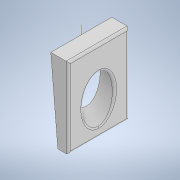
# Autodesk Inventor part: waterHeaterVent-V02
Saved by Autodesk Inventor 2021.1 (Build 251245010, 245A)
## iProperties
Created: 2020-10-25
Part Number: waterHeaterVent-V02
Material: Generic
Document SubType Name: Modeling
Designer: robst
Density: 1 g/cm^3
Appearance: Default
Author: robst
Autodesk Inventor part; units mm, degrees
ref_plane "YZ Plane" through (0, 0, 0) normal (1, 0, 0) x (0, 1, 0)
ref_plane "XZ Plane" through (0, 0, 0) normal (0, 1, 0) x (-1, 0, 0)
sketch "Sketch1" plane through (0, 0, 0) normal (0, 0, 1) x (1, 0, 0)
  line L0 (0, 0) -> (5.1111, -58.42)
  line L1 (0, -70.104) -> (0, 11.684) projected
  line L2 (0, 0) -> (12.7, 0)
  line L3 (12.7, 0) -> (12.7, -58.42)
  line L4 (5.1111, -58.42) -> (12.7, -58.42)
  dimension "d0" = 5
  dimension "d1" = 12.7
  dimension "d3" = 58.42
  constraints: 8 end point, 2 horizontal, 1 vertical
  measures "d0" angle of L0 L1
  measures "d1" distance of L0.start L2.end
  measures "d3" distance of L2.end L3.end
extrude "Extrusion1" add sketch "Sketch1" along normal mid plane 44.45
ref_plane "Work Plane1" through (12.7, -58.42, 0) normal (0.7071, -0.7071, 0) x (0, 0, 1)
sketch "Sketch2" plane through (12.7, -58.42, 0) normal (0.7071, -0.7071, 0) x (0, 0, 1)
  line L0 (22.225, 0) -> (22.225, -41.3092) projected
  line L1 (22.225, -41.3092) -> (-22.225, -41.3092) projected
  line L2 (-22.225, -41.3092) -> (-22.225, 0) projected
  line L3 (-22.225, 0) -> (22.225, 0) projected
  circle A0 centre (0, -15.9092) radius 11.43
  point P0 (0, -32.3289)
  dimension "d7" = 22.86
  dimension "d10" = 25.4
  constraints: 1 centre point
  measures "d7" diameter of A0
  measures "d10" distance from line of A0.centre L1
extrude "Extrusion2" cut sketch "Sketch2" against normal through all contours A0
sketch "Sketch3" plane through (5.1111, -58.42, -22.225) normal (-0.9962, -0.0872, 0) x (0, 0, 1)
  line L0 (0, 0) -> (0, 58.6432) construction
  line L1 (0, 7.62) -> (44.45, 7.62) construction
  line L2 (44.45, 58.6432) -> (44.45, 0) construction
  line L3 (0, 0) -> (44.45, 0) construction
  line L4 (17.7759, 11.43) -> (15.1515, 3.81)
  line L5 (15.1515, 3.81) -> (14.0585, 3.81)
  line L6 (14.0585, 3.81) -> (11.4341, 11.43)
  line L7 (11.4341, 11.43) -> (12.5209, 11.43)
  line L8 (12.5209, 11.43) -> (14.6328, 5.1006)
  line L9 (14.6328, 5.1006) -> (16.7447, 11.43)
  line L10 (16.7447, 11.43) -> (17.7759, 11.43)
  line L11 (21.166, 6.6814) -> (18.2822, 6.6814)
  line L12 (18.2822, 6.6814) -> (18.2822, 7.6077)
  line L13 (18.2822, 7.6077) -> (21.166, 7.6077)
  line L14 (21.166, 7.6077) -> (21.166, 6.6814)
  spline S0 degree 2 poles (26.9211, 7.62) (26.9211, 5.5699) (25.7293, 3.6494) (24.4882, 3.6494) knots 0 0 0 1 2 2 2
  spline S1 degree 2 poles (24.4882, 3.6494) (23.2284, 3.6494) (22.049, 5.6069) (22.049, 7.6138) knots 0 0 0 1 2 2 2
  spline S2 degree 2 poles (22.049, 7.6138) (22.049, 9.6763) (23.2408, 11.5844) (24.4882, 11.5844) knots 0 0 0 1 2 2 2
  spline S3 degree 2 poles (24.4882, 11.5844) (25.7417, 11.5844) (26.9211, 9.6084) (26.9211, 7.62) knots 0 0 0 1 2 2 2
  spline S4 degree 2 poles (25.612, 5.2982) (25.7602, 5.6749) (25.8837, 6.8358) (25.8837, 7.62) knots 0 0 0 1 2 2 2
  spline S5 degree 2 poles (25.8837, 7.62) (25.8837, 8.4042) (25.7602, 9.559) (25.6058, 9.948) knots 0 0 0 1 2 2 2
  spline S6 degree 2 poles (25.6058, 9.948) (25.4515, 10.337) (24.9142, 10.7384) (24.4882, 10.7384) knots 0 0 0 1 2 2 2
  spline S7 degree 2 poles (24.4882, 10.7384) (24.0621, 10.7384) (23.5125, 10.337) (23.3519, 9.9356) knots 0 0 0 1 2 2 2
  spline S8 degree 2 poles (23.3519, 9.9356) (23.1976, 9.5466) (23.0864, 8.361) (23.0864, 7.6138) knots 0 0 0 1 2 2 2
  spline S9 degree 2 poles (23.0864, 7.6138) (23.0864, 6.8111) (23.1852, 5.7366) (23.3458, 5.3167) knots 0 0 0 1 2 2 2
  spline S10 degree 2 poles (23.3458, 5.3167) (23.494, 4.9215) (24.0435, 4.4954) (24.4882, 4.4954) knots 0 0 0 1 2 2 2
  spline S11 degree 2 poles (24.4882, 4.4954) (24.9081, 4.4954) (25.4576, 4.8968) (25.612, 5.2982) knots 0 0 0 1 2 2 2
  line L15 (32.596, 3.81) -> (27.8968, 3.81)
  line L16 (27.8968, 3.81) -> (27.8968, 4.8906)
  spline S12 degree 2 poles (27.8968, 4.8906) (28.4031, 5.3661) (29.3047, 6.2491) (29.7369, 6.7246) knots 0 0 0 1 2 2 2
  spline S13 degree 2 poles (29.7369, 6.7246) (30.6076, 7.6818) (31.2436, 8.8303) (31.2436, 9.4416) knots 0 0 0 1 2 2 2
  spline S14 degree 2 poles (31.2436, 9.4416) (31.2436, 9.7627) (31.046, 10.2444) (30.867, 10.3988) knots 0 0 0 1 2 2 2
  spline S15 degree 2 poles (30.867, 10.3988) (30.6879, 10.5531) (30.2186, 10.7075) (29.9345, 10.7075) knots 0 0 0 1 2 2 2
  spline S16 degree 2 poles (29.9345, 10.7075) (29.6628, 10.7075) (29.1071, 10.5717) (28.8539, 10.4667) knots 0 0 0 1 2 2 2
  spline S17 degree 2 poles (28.8539, 10.4667) (28.6378, 10.3802) (28.2364, 10.1332) (28.1129, 10.0468) knots 0 0 0 1 2 2 2
  line L17 (28.1129, 10.0468) -> (28.0573, 10.0468)
  line L18 (28.0573, 10.0468) -> (28.0573, 11.1336)
  spline S18 degree 2 poles (28.0573, 11.1336) (28.3723, 11.288) (29.5023, 11.5906) (30.0086, 11.5906) knots 0 0 0 1 2 2 2
  spline S19 degree 2 poles (30.0086, 11.5906) (31.0769, 11.5906) (32.2811, 10.4605) (32.2811, 9.4972) knots 0 0 0 1 2 2 2
  spline S20 degree 2 poles (32.2811, 9.4972) (32.2811, 9.0464) (32.0711, 8.2931) (31.8859, 7.972) knots 0 0 0 1 2 2 2
  spline S21 degree 2 poles (31.8859, 7.972) (31.7006, 7.6385) (31.1634, 6.984) (30.867, 6.669) knots 0 0 0 1 2 2 2
  spline S22 degree 2 poles (30.867, 6.669) (30.3853, 6.1442) (29.2059, 5.0203) (28.8539, 4.693) knots 0 0 0 1 2 2 2
  line L19 (28.8539, 4.693) -> (32.596, 4.693)
  line L20 (32.596, 4.693) -> (32.596, 3.81)
  point P0 (22.225, 58.6432)
  dimension "d12" = 7.62
  constraints: 2 end point, 2 horizontal, 2 point on line
  measures "d12" distance between parallel lines of L3 L1
extrude "Extrusion3" cut sketch "Sketch3" against normal blind 1.27
fillet "Fillet3" radius 1.5875 5 edges at (12.7, 0, 0) (12.7, -29.21, 22.225) (12.7, -29.21, -22.225) (12.7, -58.42, 0) (12.7, -35.921, -11.43)
equation "\"d0\" = backAngle"
equation "\"d1\" = topPartDepth"
equation "\"d3\" = partHeight"
equation "\"d4\" = partWidth"
equation "\"d7\" = pipeExteriorDiameter"
equation "\"d10\" = pipeCenter"
equation "\"d13\" = textDepth"
equation "\"d16\" = filletEdge"
equation "\"topPartDepth\" = 12.7"
equation "\"backAngle\" = 5deg"
equation "\"partHeight\" = 58.42"
equation "\"partWidth\" = 44.45"
equation "\"pipeExteriorDiameter\" = 22.86"
equation "\"pipeCenter\" = 25.4"
equation "\"filletEdge\" = 1.5875"
equation "\"textDepth\" = 1.27"
body "Solid1"
